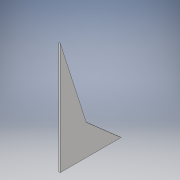
# Autodesk Inventor part: fins
Saved by Autodesk Inventor 2017 (Build 210142000, 142)
## iProperties
Created: 2017-04-26
Part Number: fins
Material: Generic
Document SubType Name: Modeling
Designer: seane
Density: 1 g/cm^3
Appearance: Default
Author: seane
Autodesk Inventor part; units mm, degrees
ref_plane "YZ Plane" through (0, 0, 0) normal (1, 0, 0) x (0, 1, 0)
ref_plane "XZ Plane" through (0, 0, 0) normal (0, 1, 0) x (-1, 0, 0)
ref_plane "XY Plane" through (0, 0, 0) normal (0, 0, 1) x (1, 0, 0)
sketch "Sketch1" plane through (0, 0, 0) normal (1, 0, 0) x (0, 1, 0)
  line L0 (0, 0) -> (0, -63.5)
  line L1 (0, 0) -> (63.5, 0) construction
  line L2 (0, 0) -> (116.84, 0)
  line L3 (116.84, 0) -> (31.75, -27.202)
  line L4 (31.75, -27.202) -> (0, -63.5)
  dimension "d5" = 63.5
  dimension "d6" = 90
  dimension "d7" = 116.84
  constraints: 10 end point, 2 horizontal, 1 perpendicular, 1 vertical
  measures "d5" distance of L0.start L0.end
  measures "d6" angle of L0 L1
  measures "d7" distance of L0.start L2.end
extrude "Extrusion1" add sketch "Sketch1" along normal blind 1.27
body "Solid1"
